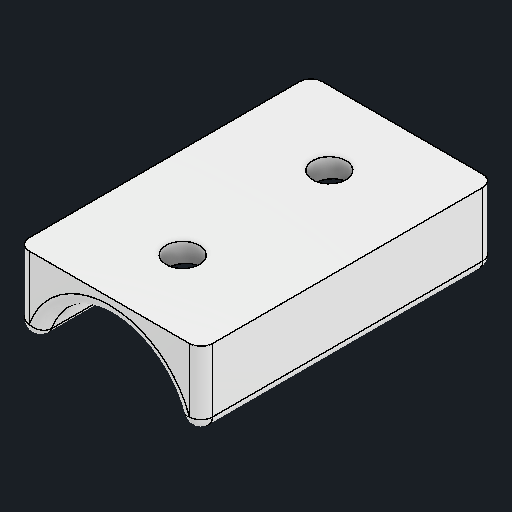
# Autodesk Inventor part: Pipe Adapter
Saved by Autodesk Inventor 2026.2 (Build 302298000, 298)
## iProperties
Created: 2026-10-01
Part Number: Pipe Adapter
Material: ABS Plastic
Document SubType Name: Modeling
Designer: Joshua Eah
Density: 1.06 g/cm^3
Appearance: Smooth - White
Mass: 12.0594 g
Surface Area: 52.5314 cm^2
Volume: 11.3767 cm^3
Author: Joshua Eah
Autodesk Inventor part; units mm, degrees
ref_plane "YZ Plane" through (0, 0, 0) normal (1, 0, 0) x (0, 1, 0)
ref_plane "XZ Plane" through (0, 0, 0) normal (0, 1, 0) x (-1, 0, 0)
ref_plane "XY Plane" through (0, 0, 0) normal (0, 0, 1) x (1, 0, 0)
sketch "Sketch1" plane through (0, 0, 0) normal (0, 0, 1) x (1, 0, 0)
  circle A0 centre (0, 0) radius 12.7
  line L0 (-15.875, 15.875) -> (15.875, 15.875)
  line L1 (15.875, 15.875) -> (15.875, -15.875)
  line L2 (15.875, -15.875) -> (-15.875, -15.875)
  line L3 (-15.875, -15.875) -> (-15.875, 15.875)
  line L4 (-15.875, 15.875) -> (15.875, -15.875) construction
  line L5 (15.875, 15.875) -> (-15.875, -15.875) construction
  line L6 (-15.875, 0) -> (15.875, 0)
  point P0 (-12.7, 0)
  point P1 (12.7, 0)
  dimension "d0" = 25.4
  dimension "d1" = 31.75
  dimension "d2" = 31.75
  constraints: 14 end point, 4 midpoint, 2 parallel, 1 centre point, 1 coincident, 1 horizontal, 1 perpendicular
  measures "d0" diameter of A0
  measures "d1" distance of L1.end L2.end
  measures "d2" distance of L0.end L1.end
extrude "Extrusion1" add sketch "Sketch1" along normal blind 50.8 contours A0 L6 L3 L0 L1
sketch "Sketch2" plane through (-15.875, 15.875, 0) normal (0, 1, 0) x (1, 0, 0)
  line L0 (31.75, 0) -> (0, 0) construction
  line L1 (0, 0) -> (0, -50.8) construction
  line L2 (31.75, -50.8) -> (0, -50.8) construction
  line L3 (31.75, 0) -> (31.75, -50.8) construction
  line L4 (15.875, -50.8) -> (15.875, 0)
  point P0 (15.875, -38.1)
  point P1 (15.875, -12.7)
  point P2 (15.875, -25.4)
  dimension "d7" = 25.4
  dimension "d8" = 25.4
  constraints: 3 midpoint, 2 end point, 2 point on line
  measures "d7" distance of point (15.875, -38.1) point (15.875, -12.7)
  measures "d8" diameter of point (15.875, -38.1) point (15.875, -25.4)
hole "Hole1" at (0, 15.875, 38.1) at (0, 15.875, 12.7) direction (0, -1, 0) diameter 5.7912 end through all clearance for "Flat Head Machine Screw (82)" size "#12" standard "Ansi Unified Screw Threads"
fillet "Fillet1" radius 2 4 edges at (15.875, 0, 25.4) (12.7, 0, 25.4) (-15.875, 0, 25.4) (-12.7, 0, 25.4)
fillet "Fillet2" radius 2 10 edges at (-14.2101, 2.8831, 50.8) (0, 12.7, 50.8) (14.2101, 2.8831, 50.8) (15.875, 10.3649, 50.8) (-15.875, 10.3649, 50.8) (-14.2101, 2.8831, 0) (0, 12.7, 0) (14.2101, 2.8831, 0) (15.875, 10.3649, 0) (-15.875, 10.3649, 0)
equation "\"d0\" = tubeOD"
equation "\"d3\" = attachmentLength"
equation "\"d8\" = d7"
equation "\"tubeOD\" = 25.4"
equation "\"attachmentLength\" = 50.8"
body "Solid1"
